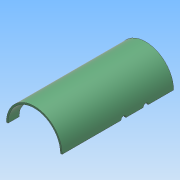
# Autodesk Inventor part: Timing_PVC Pipe
Saved by Autodesk Inventor 2018.1 (Build 221171000, 171)
## iProperties
Created: 2019-02-11
Part Number: Timing_PVC Pipe
Material: Generic
Document SubType Name: Modeling
Designer: James
Density: 1 g/cm^3
Appearance: Default
Author: James
Autodesk Inventor part; units mm, degrees
ref_plane "YZ Plane" through (0, 0, 0) normal (1, 0, 0) x (0, 1, 0)
ref_plane "XZ Plane" through (0, 0, 0) normal (0, 1, 0) x (-1, 0, 0)
ref_plane "XY Plane" through (0, 0, 0) normal (0, 0, 1) x (1, 0, 0)
sketch "Sketch1" plane through (0, 0, 0) normal (0, 1, 0) x (-1, 0, 0)
  circle A0 centre (0, 0) radius 25
  circle A1 centre (0, 0) radius 23.5
  dimension "d0" = 1.5
  dimension "d27" = 50
  constraints: 2 centre point, 2 coincident
  measures "d0" radial gap between concentric circles of A0 A1
  measures "d27" diameter of A0
extrude "Extrusion1" add sketch "Sketch1" along normal blind 100
sketch "Sketch2" plane through (0, 0, 0) normal (0, 0, 1) x (1, 0, 0)
  line L0 (-25, 85) -> (0, 85)
  line L1 (0, 85) -> (0, 10)
  line L2 (0, 10) -> (-25, 10)
  line L3 (-25, 10) -> (-25, 85)
  line L4 (25, 100) -> (-25, 100) projected
  line L5 (-25, 0) -> (25, 0) projected
  point P0 (0, 0)
  dimension "d4" = 75
  dimension "d5" = 10
  constraints: 8 end point, 2 parallel, 1 horizontal, 1 perpendicular, 1 vertical alignment
  measures "d4" distance of L2.end L0.start
  measures "d5" distance between parallel lines of L5 L2
extrude "Extrusion2" cut sketch "Sketch2" along normal mid plane 20
fillet "Fillet1" radius 5 4 edges at (-22.0895, 85, -10) (-22.0895, 85, 10) (-22.0895, 10, 10) (-22.0895, 10, -10)
sketch "Sketch3" plane through (0, 0, 0) normal (1, 0, 0) x (0, 1, 0)
  line L0 (-17, 0) -> (102, 0) projected
  line L1 (85, -5) -> (85, 5) projected
  point P0 (0, 0)
  point P1 (75, 0)
  point P2 (55, 0)
  dimension "d9" = 20
  dimension "d10" = 10
  constraints: 1 horizontal alignment, 1 point on line
  measures "d9" distance of point (55, 0) point (75, 0)
  measures "d10" distance from line of point (75, 0) L1
hole "Hole1" at (0, 75, 0) at (0, 55, 0) direction (1, 0, 0) diameter 4.5 end through all clearance for "Socket Head Cap Screw" size "M4" standard "Ansi Metric M Profile"
sketch "Sketch4" plane through (0, 100, 0) normal (0, 1, 0) x (1, 0, 0)
  circle A0 centre (0, 0) radius 25 projected
  line L0 (26, 27) -> (-26, 27)
  line L1 (-26, 27) -> (-26, 0)
  line L2 (-26, 0) -> (26, 0)
  line L3 (26, 0) -> (26, 27)
  dimension "d21" = 50
  dimension "d22" = 27
  dimension "d23" = 52
  dimension "d24" = 26
  constraints: 8 end point, 2 parallel, 1 horizontal, 1 horizontal alignment, 1 perpendicular
  measures "d21" diameter of A0
  measures "d22" distance of L2.end L0.start
  measures "d23" distance of L0.start L0.end
  measures "d24" distance from line of A0.centre L3
extrude "Extrusion3" cut sketch "Sketch4" against normal through all contours L2 A0 | A0 L2 L1 L0 L3 picked at (-4.8086, 15.3121)
equation "\"d24\" = 0.5 * d23"
body "Solid1"
